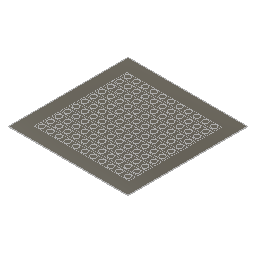
WordClock-Frame (Autodesk Fusion 360 design; units mm, degrees)
Autodesk Fusion 360 part; units mm, degrees
sketch "Sketch2" plane through (0, 0, 0) normal (0, 0, 1) x (1, 0, 0)
  line L0 (0, 0) -> (16.6, 0)
  line L1 (16.6, 0) -> (16.6, 10.5)
  line L2 (16.6, 10.5) -> (0, 10.5)
  line L3 (0, 10.5) -> (0, 0)
  line L4 (5.7, 2.25) -> (10.9, 2.25)
  line L5 (10.9, 2.25) -> (10.9, 8.25)
  line L6 (10.9, 8.25) -> (5.7, 8.25)
  line L7 (5.7, 8.25) -> (5.7, 2.25)
  line L8 (5.7, 2.25) -> (10.9, 8.25) construction
  line L9 (0, 10.5) -> (16.6, 0) construction
  circle A0 centre (10.9, 5.25) radius 3
  dimension "d6" = 16.6
  dimension "d7" = 10.5
  dimension "d8" = 6
  dimension "d9" = 5.2
  dimension "d10" = 6
  constraint horizontal L0
  constraint vertical L1
  constraint horizontal L2
  constraint vertical L3
  constraint coincident L0.start L3.end
  constraint horizontal L4
  constraint vertical L5
  constraint horizontal L6
  constraint vertical L7
  constraint midpoint L8 L9
  constraint midpoint L5 A0.centre
  measures "d6" distance of L1.end L2.end
  measures "d7" distance of L0.start L2.end
  measures "d8" distance of L4.end L5.end
  measures "d9" distance of L4.start L4.end
  measures "d10" diameter of A0
extrude "Extrude1" add sketch "Sketch2" against normal blind 1 contours L0 L1 L2 L3 | L4 L6 L7 A0 | L5 A0 | L5 A0 makes body 1
extrude "Extrude2" add sketch "Sketch2" along normal blind 2.2 contours L4 L6 L7 A0 | L5 A0 picked at (9.035, 5.3247) bodies 1
extrude "Extrude3" add sketch "Sketch2" along normal blind 1.1 contours L5 A0 picked at (12.1183, 6.0057) bodies 1
sketch "Sketch3" plane through (0, 0, -1) normal (0, 0, -1) x (1, 0, 0)
  line L0 (0, 0) -> (0, -10.5)
  line L1 (0, -10.5) -> (16.6, -10.5)
  line L2 (16.6, -10.5) -> (16.6, 0)
  line L3 (16.6, 0) -> (0, 0)
  line L4 (0, 1) -> (16.6, 1)
  line L5 (16.6, 1) -> (16.6, -11.5)
  line L6 (16.6, -11.5) -> (0, -11.5)
  line L7 (0, -11.5) -> (0, 1)
  line L8 (0, 0) -> (16.6, -10.5) construction
  line L9 (16.6, 1) -> (0, -11.5) construction
  dimension "d18" = 16.6
  dimension "d19" = 12.5
  constraint horizontal L4
  constraint vertical L5
  constraint horizontal L6
  constraint vertical L7
  constraint coincident L0.start L3.end
  constraint coincident L1.end L2.start
  constraint midpoint L8 L9
  measures "d18" distance of L4.start L4.end
  measures "d19" distance of L4.start L6.end
extrude "Extrude4" add sketch "Sketch3" against normal blind 5.5 separate body makes body 2
combine "Combine1" operation cut target body 2 tool bodies 1
sketch "Sketch5" plane through (0, 0, 2.2) normal (0, 0, -1) x (1, 0, 0)
  line L0 (5.7, -2.25) -> (5.7, -8.25)
  line L1 (5.7, -8.25) -> (10.9, -8.25)
  line L2 (10.9, -8.25) -> (10.9, -2.25)
  line L3 (10.9, -2.25) -> (5.7, -2.25)
sketch "Sketch6" plane through (0, 0, 2.2) normal (0, 0, -1) x (1, 0, 0)
  line L0 (5.6, -2.5) -> (11, -7.9) construction
  circle A0 centre (8.3, -5.2) radius 2.5
  dimension "d23" = 5
  constraint midpoint L0 A0.centre
  measures "d23" diameter of A0
extrude "Extrude5" cut sketch "Sketch6" against normal up to surface (2.8 mm away) draft 45 from surface at 0.5 bodies 2
sketch "Sketch7" plane through (0, 0, 4.5) normal (0, 0, 1) x (-1, 0, 0)
  circle A0 centre (-8.3, -5.2) radius 5.3
  line L0 (-16.6, -11.5) -> (0, -11.5)
  line L1 (0, -11.5) -> (0, 1)
  line L2 (0, 1) -> (-16.6, 1)
  line L3 (-16.6, 1) -> (-16.6, -11.5)
  line L4 (0, -11.5) -> (-16.6, 1) construction
  line L5 (0, -13.55) -> (-16.6, -13.55)
  line L6 (-16.6, -13.55) -> (-16.6, 3.05)
  line L7 (-16.6, 3.05) -> (0, 3.05)
  line L8 (0, 3.05) -> (0, -13.55)
  line L9 (-16.6, -13.55) -> (0, 3.05) construction
  dimension "d27" = 16.6
  dimension "d28" = 16.6
  constraint coincident L0.end L1.start
  constraint coincident L2.end L3.start
  constraint horizontal L5
  constraint vertical L6
  constraint horizontal L7
  constraint vertical L8
  constraint midpoint L4 L9
  measures "d27" distance of L5.start L5.end
  measures "d28" distance of L5.end L6.end
extrude "Extrude6" add sketch "Sketch7" against normal blind 1 contours L0 L5 L6 L8 | L2 L6 L7 L8 bodies 2
extrude "Extrude8" add sketch "Sketch7" against normal blind 0.2 contours A0 | L0 L1 L2 L3 L6 L8 bodies 2
sketch "Sketch8" plane through (16.6, 0, 0) normal (1, 0, 0) x (0, 1, 0)
  line L0 (13.55, 4.5) -> (-3.05, 4.5)
  line L1 (-3.05, 4.5) -> (-3.05, 3.5)
  line L2 (-3.05, 3.5) -> (-1, 3.5)
  line L3 (0, 0) -> (10.5, 0)
  line L4 (11.5, 3.5) -> (13.55, 3.5)
  line L5 (13.55, 3.5) -> (13.55, 4.5)
  line L6 (5.25, 4.5) -> (5.25, -1.3) construction
  line L7 (11.5, -1) -> (10.5, -1)
  line L8 (10.2, -1.3002) -> (10.2001, -1.3999)
  line L9 (10.2001, -1.3999) -> (11.2, -1.3999)
  line L10 (11.5, -1.0999) -> (11.5, -1)
  arc A0 (11.2, -1.3999) -> (11.5, -1.0999) centre (11.2, -1.0999) ccw
  arc A1 (10.5, -1) -> (10.2, -1.3002) centre (10.5, -1.3) ccw
  arc A2 (-1, -1.0999) -> (-0.7, -1.3999) centre (-0.7, -1.0999) ccw
  line L11 (0.2999, -1.3999) -> (-0.7, -1.3999)
  line L12 (0.3, -1.3002) -> (0.2999, -1.3999)
  arc A3 (0.3, -1.3002) -> (0, -1) centre (0, -1.3) ccw
  line L13 (-1, -1.0999) -> (-1, -1)
  line L14 (-1, -1) -> (0, -1)
  line L15 (10.5, 0) -> (10.5, -1)
  dimension "d39" = 16.6
  dimension "d73" = 0.3
  dimension "d74" = 0.3
  dimension "d77" = 0.4
  dimension "d78" = 0.8
  constraint midpoint L0 L6.start
  constraint perpendicular L3 L6
  constraint horizontal L7
  constraint horizontal L9
  constraint vertical L10
  constraint tangent L9 A0
  constraint tangent L10 A0
  constraint tangent L7 A1
  constraint tangent L8 A1
  constraint symmetric L6 L7.start L13.end
  constraint symmetric L6 L8.end L11.start
  constraint symmetric L6 L9.end A2.end
  constraint symmetric L6 L10.start A2.start
  constraint symmetric L6 A0 A2
  constraint symmetric L6 L7.end A3.end
  constraint symmetric L6 L8.start L12.start
  constraint symmetric L6 A1 A3
  measures "d39" distance of L1 L5
  measures "d73" radius of A0
  measures "d74" radius of A1
  measures "d77" distance of L7 L9
extrude "Extrude11" add sketch "Sketch8" against normal up to surface (16.6 mm away) bodies 2
pattern_linear "R-Pattern1" count 11 spacing 16.6 along (1, 0, 0) of bodies 2 makes body 3 at (22.1333, 2.4833, 4.5) makes body 4 at (44.2667, 8.0167, 4.5) makes body 5 at (55.3333, 2.4833, 4.5) makes body 6 at (77.4667, 8.0167, 4.5) makes body 7 at (94.0667, 8.0167, 4.5) makes body 8 at (105.1333, 2.4833, 4.5) makes body 9 at (121.7333, 2.4833, 4.5) makes body 10 at (138.3333, 2.4833, 4.5) makes body 11 at (154.9333, 2.4833, 4.5) makes body 12 at (171.5333, 2.4833, 4.5)
combine "Combine2" operation add target body 2 tool bodies 3 4 5 6 7 8 9 10 11 12
pattern_linear "R-Pattern2" count 1 spacing 0 along (1, 0, 0) count 11 spacing 16.6 along (0, -1, 0) of bodies 2 makes body 13 at (60.8667, -14.1167, 4.5) makes body 14 at (60.8667, -30.7167, 4.5) makes body 15 at (60.8667, -47.3167, 4.5) makes body 16 at (60.8667, -63.9167, 4.5) makes body 17 at (60.8667, -80.5167, 4.5) makes body 18 at (60.8667, -97.1167, 4.5) makes body 19 at (60.8667, -113.7167, 4.5) makes body 20 at (60.8667, -130.3167, 4.5) makes body 21 at (60.8667, -146.9167, 4.5) makes body 22 at (60.8667, -163.5167, 4.5)
combine "Combine3" operation add target body 2 tool bodies 13 14 15 16 17 18 19 20 21 22
sketch "Sketch9" plane through (0, 0, 4.5) normal (0, 0, 1) x (-1, 0, 0)
  line L0 (-182.6, -13.55) -> (0, -13.55)
  line L1 (0, -13.55) -> (0, 169.05)
  line L2 (0, 169.05) -> (-182.6, 169.05)
  line L3 (-182.6, 169.05) -> (-182.6, -13.55)
  line L4 (0, -13.55) -> (-182.6, 169.05) construction
  line L5 (23.7, -37.25) -> (-206.3, -37.25)
  line L6 (-206.3, -37.25) -> (-206.3, 192.75)
  line L7 (-206.3, 192.75) -> (23.7, 192.75)
  line L8 (23.7, 192.75) -> (23.7, -37.25)
  line L9 (-206.3, -37.25) -> (23.7, 192.75) construction
  line L10 (-5.7, 14.35) -> (-5.7, 8.35)
  line L11 (-171.7, 14.35) -> (-171.7, 8.35)
  line L12 (-22.3, -8.25) -> (-27.5, -8.25)
  line L13 (-22.3, 157.75) -> (-27.5, 157.75)
  dimension "d63" = 230
  dimension "d64" = 230
  dimension "d67" = 23.7
  dimension "d68" = 23.7
  dimension "d69" = 23.7
  dimension "d70" = 23.7
  dimension "d79" = 166
  dimension "d80" = 166
  constraint coincident L0.end L1.start
  constraint coincident L2.end L3.start
  constraint horizontal L5
  constraint vertical L6
  constraint horizontal L7
  constraint vertical L8
  constraint midpoint L4 L9
  measures "d63" distance of L5.start L5.end
  measures "d64" distance of L5.end L6.end
  measures "d67" distance of L1 L8
  measures "d68" distance of L3 L6
  measures "d69" distance of L0 L5
  measures "d70" distance of L2 L7
  measures "d79" distance of L10 L11
  measures "d80" distance of L12 L13
extrude "Extrude10" add sketch "Sketch9" against normal blind 1 bodies 2
equation "strip = 16.6 mm"
equation "stripWidth = 10.5 mm"
equation "ledWidth = 6 mm"
equation "ledHeight = 2.2 mm"
equation "stripBorder = stripWidth + 2 mm"
equation "d6 = strip"
equation "d7 = stripWidth"
equation "d8 = ledWidth"
equation "d9 = ledLength"
equation "d10 = ledWidth"
equation "stripHeight = 1 mm"
equation "d12 = -stripHeight"
equation "d14 = ledHeight"
equation "d16 = ledHeight / 2"
equation "d18 = strip"
equation "d19 = stripBorder"
equation "stripBlockHeight = 5.5 mm"
equation "d21 = -stripBlockHeight"
equation "d27 = strip"
equation "d28 = strip"
equation "flat = 1 mm"
equation "d30 = -flat"
equation "firstLayer = 0.2 mm"
equation "d35 = -firstLayer"
equation "d57 = strip"
equation "d62 = strip"
equation "d72 = -flat"
equation "ledLength = 5.2 mm"
